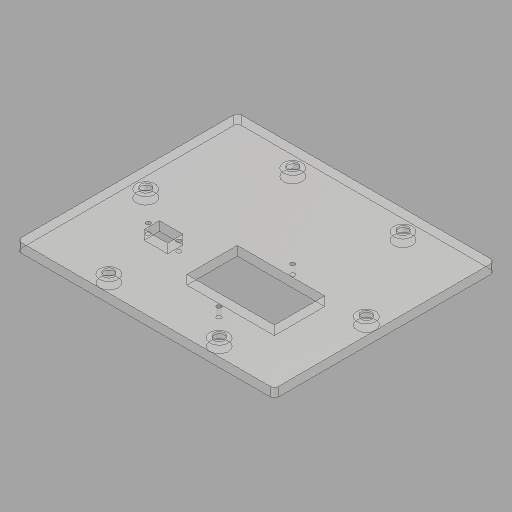
# Autodesk Inventor part: BT701_trajan20_21
Saved by Autodesk Inventor 2023 (Build 270158000, 158)
## iProperties
Company: HTBLA Kaindorf
RuleStatus: InUse
AfterDocNew0: iProperties-Editor_aufrufen
Created: 2022-08-21
Part Number: BT701_trajan20_21
Project: Zeichenmaschine_v2
Material: Acryl
Description: Plexi_100x80
Document SubType Name: Modeling
Designer: trajan20
Density: 1.188 g/cm^3
Appearance: Transparent - farblos
Mass: 88.8642 g
Surface Area: 350.035 cm^2
Volume: 74.8015 cm^3
Author: jan
Keywords: 2021
Autodesk Inventor part; units mm, degrees
ref_plane "YZ Plane" through (0, 0, 0) normal (1, 0, 0) x (0, 1, 0)
ref_plane "XZ Plane" through (0, 0, 0) normal (0, 1, 0) x (-1, 0, 0)
ref_plane "XY Plane" through (0, 0, 0) normal (0, 0, 1) x (1, 0, 0)
derived "BT000_trajan20_22_Zeichenmaschine_neu_Masterskizze.ipt"
sketch "Skizze3" plane through (0, 0, 0) normal (0, 0, 1) x (1, 0, 0)
  line L0 (0, 0) -> (-120, 0)
  line L1 (-120, 0) -> (-120, 140)
  line L2 (-120, 140) -> (0, 140)
  line L3 (0, 140) -> (0, 0)
  line L4 (-120, 140) -> (0, 140)
  line L5 (-39.5, 29.6) -> (-47.9, 29.6)
  line L6 (-47.9, 29.6) -> (-47.9, 42.4)
  line L7 (-47.9, 42.4) -> (-39.5, 42.4)
  line L8 (-39.5, 42.4) -> (-39.5, 29.6)
  line L9 (-30, 62.4) -> (-57.4, 62.4)
  line L10 (-57.4, 62.4) -> (-57.4, 110)
  line L11 (-57.4, 110) -> (-30, 110)
  line L12 (-30, 110) -> (-30, 62.4)
  point P0 (-10, 40)
  point P1 (-10, 100)
  point P2 (-110, 40)
  point P3 (-110, 100)
  point P4 (-60, 10)
  point P5 (-60, 130)
  point P6 (-60, 140)
  point P7 (-120, 70)
  point P8 (-23.65, 86.2)
  point P9 (-63.75, 86.2)
  point P10 (-30, 86.2)
  point P11 (-57.4, 86.2)
  point P12 (-43.7, 42.4)
  point P13 (-43.7, 62.4)
  point P14 (-43.7, 27.65)
  point P15 (-43.7, 44.35)
  point P16 (-43.7, 29.6)
  dimension "d4" = 140
  dimension "d5" = 120
  dimension "d19" = 10
  dimension "d20" = 10
  dimension "d21" = 10
  dimension "d22" = 10
  dimension "d23" = 40
  dimension "d24" = 40
  dimension "d34" = 8.4
  dimension "d35" = 12.8
  dimension "d36" = 47.6
  dimension "d37" = 27.4
  dimension "d43" = 6.35
  dimension "d44" = 6.35
  dimension "d53" = 30
  dimension "d54" = 20
  dimension "d55" = 30
  dimension "d56" = 1.95
  dimension "d57" = 1.95
  constraints: 26 end point, 7 midpoint, 7 vertical alignment, 6 parallel, 4 horizontal, 4 horizontal alignment, 3 perpendicular
  measures "d4" distance between parallel lines of L2 L0
  measures "d5" distance between parallel lines of L1 L3
  measures "d19" distance from line of L3 point (-10, 40)
  measures "d20" distance from line of L1 point (-110, 40)
  measures "d21" distance from line of L0 point (-60, 10)
  measures "d22" distance from line of L2 point (-60, 130)
  measures "d23" distance from line of L2 point (-110, 100)
  measures "d24" distance from line of L0 point (-110, 40)
  measures "d34" distance between parallel lines of L6 L8
  measures "d35" distance between parallel lines of L5 L7
  measures "d36" distance between parallel lines of L9 L11
  measures "d37" distance between parallel lines of L10 L12
  measures "d43" distance from line of L12 point (-23.65, 86.2)
  measures "d44" distance from line of point (-63.75, 86.2) L10
  measures "d53" distance between parallel lines of L2 L11
  measures "d54" distance between parallel lines of L9 L7
  measures "d55" distance between parallel lines of L12 L3
  measures "d56" distance from line of L7 point (-43.7, 44.35)
  measures "d57" distance from line of point (-43.7, 27.65) L5
extrude "Extrusion3" add sketch "Skizze3" along normal blind 5
fillet "Rundung3" radius 2 4 edges at (0, 0, 2.5) (0, 140, 2.5) (-120, 140, 2.5) (-120, 0, 2.5)
hole "Bohrung1" at (-10, 40, 0) at (-10, 100, 0) at (-110, 40, 0) at (-110, 100, 0) at (-60, 10, 0) at (-60, 130, 0) direction (0, 0, 1) diameter 5.5 end through all counterbore diameter 10 counterbore depth 4
hole "Bohrung2" at (-23.65, 86.2, 0) at (-63.75, 86.2, 0) at (-43.7, 27.65, 0) at (-43.7, 44.35, 0) direction (0, 0, 1) diameter 2.459 end through all thread size "M3x0.5" class "6H" standard "ISO Metric profile"
equation "\"d4\" = Basis_Haupt_Breite_Profillänge + 4 * AluProfil_Abstand"
equation "\"d5\" = Basis_Haupt_Höhe_Profillänge"
equation "\"d19\" = AluProfil_Abstand"
equation "\"d20\" = AluProfil_Abstand"
equation "\"d21\" = AluProfil_Abstand"
equation "\"d22\" = AluProfil_Abstand"
equation "\"d24\" = d23"
equation "\"d44\" = d43"
equation "\"d57\" = d56"
equation "\"Basis_Haupt_Breite_Profillänge\" = 100"
equation "\"AluProfil_Abstand\" = 10"
equation "\"Basis_Haupt_Höhe_Profillänge\" = 120"
